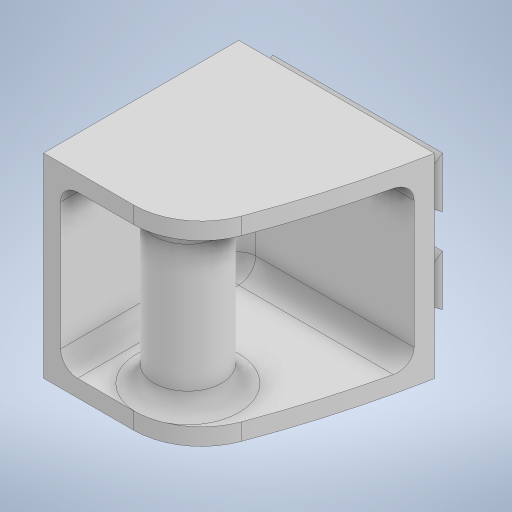
# Autodesk Inventor part: sides_fp13
Saved by Autodesk Inventor 2023 (Build 270158000, 158)
## iProperties
Created: 2023-02-13
Part Number: sides_fp13
Material: Generic
Document SubType Name: Modeling
Designer: tdal0
Density: 1 g/cm^3
Appearance: Default
Author: tdal0
Autodesk Inventor part; units mm, degrees
ref_plane "YZ Plane" through (0, 0, 0) normal (1, 0, 0) x (0, 1, 0)
ref_plane "XZ Plane" through (0, 0, 0) normal (0, 1, 0) x (-1, 0, 0)
ref_plane "XY Plane" through (0, 0, 0) normal (0, 0, 1) x (1, 0, 0)
sketch "Sketch12" plane through (0, 0, 0) normal (0, 1, 0) x (-1, 0, 0)
  line L0 (0, 0) -> (0, -102.5) construction
  line L1 (0, 0) -> (0, 102.5) construction
  line L2 (0, 102.5) -> (125, 102.5) construction
  line L3 (125, 102.5) -> (125, -102.5) construction
  line L4 (125, -102.5) -> (0, -102.5) construction
  line L5 (0, -102.5) -> (0, 102.5) construction
  line L6 (0, 102.5) -> (45, 102.5) construction
  line L7 (45, 102.5) -> (45, -102.5) construction
  line L8 (45, -102.5) -> (0, -102.5) construction
  line L9 (0, -102.5) -> (0, 102.5) construction
  line L10 (125, 0) -> (125, -217.5) construction
  line L11 (125, -217.5) -> (72.0108, -217.5) construction
  line L12 (45, -217.5) -> (45, -102.5) construction
  line L13 (125, 0) -> (125, 217.5) construction
  line L14 (125, 217.5) -> (72.0108, 217.5) construction
  line L15 (45, 217.5) -> (45, 102.5) construction
  arc A0 (34.5307, 191.4729) -> (34.5307, -191.4729) centre (548.125, 0) ccw construction
  arc A1 (34.5307, -191.4729) -> (72.0108, -217.5) centre (72.0108, -177.5) ccw construction
  arc A2 (72.0108, 217.5) -> (34.5307, 191.4729) centre (72.0108, 177.5) ccw construction
  line L16 (125, 102.5) -> (125, 107.5) construction
  line L17 (125, 217.5) -> (125, 102.5)
  line L18 (125, 102.5) -> (9.6691, 102.5)
  line L19 (125, 102.5) -> (125, 112.5) construction
  line L20 (125, 112.5) -> (11.6693, 112.5) construction
  line L21 (125, 217.5) -> (115, 217.5) construction
  line L22 (115, 217.5) -> (115, 102.5) construction
  line L23 (115, 217.5) -> (125, 217.5)
  line L24 (115, 217.5) -> (115, 112.5)
  line L25 (115, 112.5) -> (11.6693, 112.5)
  arc A3 (11.6693, 112.5) -> (9.6691, 102.5) centre (548.125, 0) ccw
  dimension "d616" = 102.5
  dimension "d617" = 102.5
  dimension "d618" = 125
  dimension "d619" = 45
  dimension "d620" = 217.5
  dimension "d621" = 217.5
  dimension "d622" = 40
  dimension "d650" = 10
  dimension "d651" = 10
  constraints: 52 end point, 13 point on circle, 12 point on line, 7 perpendicular, 4 centre point, 4 collinear, 4 parallel, 4 tangent, 3 vertical, 2 horizontal, 1 equal radius, 1 midpoint
  measures "d616" distance of L0.start L0.end
  measures "d617" distance of L0.start L1.end
  measures "d618" distance of L3.end L4.end
  measures "d619" distance of L7.end L8.end
  measures "d620" distance of L10.start L10.end
  measures "d621" distance of L10.start L13.end
  measures "d622" radius of A1
  measures "d650" distance of L2.end L19.end
  measures "d651" distance of L13.end L21.end
extrude "Extrusion12" add sketch "Sketch12" along normal blind 115
sketch "Sketch66" plane through (0, 115, 0) normal (0, 1, 0) x (1, 0, 0)
  line L0 (0, 0) -> (0, 102.5) construction
  line L1 (0, 0) -> (0, -102.5) construction
  line L2 (0, -102.5) -> (-125, -102.5) construction
  line L3 (-125, -102.5) -> (-125, 102.5) construction
  line L4 (-125, 102.5) -> (0, 102.5) construction
  line L5 (0, 102.5) -> (0, -102.5) construction
  line L6 (0, -102.5) -> (-45, -102.5) construction
  line L7 (-45, -102.5) -> (-45, 102.5) construction
  line L8 (-45, 102.5) -> (0, 102.5) construction
  line L9 (0, 102.5) -> (0, -102.5) construction
  line L10 (-125, 0) -> (-125, 217.5) construction
  line L11 (-125, 217.5) -> (-72.0108, 217.5) construction
  line L12 (-45, 217.5) -> (-45, 102.5) construction
  line L13 (-125, 0) -> (-125, -217.5) construction
  line L14 (-125, -217.5) -> (-72.0108, -217.5)
  line L15 (-45, -217.5) -> (-45, -102.5) construction
  line L16 (-120, -107.5) -> (-10.645, -107.5) construction
  arc A0 (-34.5307, -191.4729) -> (-34.5307, 191.4729) centre (-548.125, 0) ccw
  arc A1 (-72.0108, -217.5) -> (-34.5307, -191.4729) centre (-72.0108, -177.5) ccw
  arc A2 (-34.5307, 191.4729) -> (-72.0108, 217.5) centre (-72.0108, 177.5) ccw construction
  line L17 (-125, -217.5) -> (-120, -217.5) projected
  line L18 (-120, -217.5) -> (-120, -107.5)
  line L19 (-120, -217.5) -> (-120, -107.5) projected
  line L20 (-120, -107.5) -> (-10.645, -107.5)
  dimension "d643" = 102.5
  dimension "d644" = 102.5
  dimension "d645" = 125
  dimension "d646" = 45
  dimension "d647" = 217.5
  dimension "d648" = 217.5
  dimension "d649" = 40
  constraints: 36 end point, 9 point on circle, 7 perpendicular, 5 equal length, 4 point on line, 4 tangent, 3 centre point, 3 vertical, 2 horizontal, 1 equal radius, 1 midpoint
  measures "d643" distance of L0.start L0.end
  measures "d644" distance of L0.start L1.end
  measures "d645" distance of L3.end L4.end
  measures "d646" distance of L7.end L8.end
  measures "d647" distance of L10.start L10.end
  measures "d648" distance of L10.start L13.end
  measures "d649" radius of A1
extrude "Extrusion51" add sketch "Sketch66" against normal blind 10
sketch "Sketch67" plane through (0, 0, 0) normal (0, -1, 0) x (1, 0, 0)
  line L0 (-125, 217.5) -> (-72.0108, 217.5) projected
  line L1 (-120, 217.5) -> (-120, 107.5)
  arc A0 (-11.6693, 112.5) -> (-34.5307, 191.4729) centre (-548.125, 0) ccw projected
  line L2 (-120, 107.5) -> (-10.645, 107.5)
  line L3 (-120, 217.5) -> (-72.0108, 217.5)
  arc A1 (-34.5307, 191.4729) -> (-72.0108, 217.5) centre (-72.0108, 177.5) ccw projected
  arc A2 (-34.5307, 191.4729) -> (-72.0108, 217.5) centre (-72.0108, 177.5) ccw
  arc A3 (-9.6691, 102.5) -> (-10.645, 107.5) centre (-548.125, 0) ccw construction
  arc A4 (-10.645, 107.5) -> (-34.5307, 191.4729) centre (-548.125, 0) ccw
  point P0 (-105, 112.5)
  constraints: 6 end point, 4 point on circle, 2 centre point, 1 concentric, 1 perpendicular, 1 point on line, 1 vertical
extrude "Extrusion52" add sketch "Sketch67" against normal blind 10
sketch "Sketch79" plane through (0, 10, 0) normal (0, 1, 0) x (1, 0, 0)
  arc A0 (-72.0093, -220) -> (-34.5299, -193.9747) centre (-72.0093, -180) ccw construction
  circle A1 centre (-70, -187.5) radius 20
  line L0 (-120, -220) -> (-120, -107.5) projected
  line L1 (-115, -217.5) -> (-72.0108, -217.5) projected
  point P0 (0, 0)
  point P1 (-72.0093, -180)
  point P2 (-49.1947, -212.8557)
  dimension "d578" = 40
  dimension "d586" = 50
  dimension "d652" = 30
  constraints: 1 centre point, 1 coincident, 1 point on circle
  measures "d578" diameter of A1
  measures "d586" distance from line of L0 A1.centre
  measures "d652" distance from line of L1 A1.centre
extrude "Extrusion61" add sketch "Sketch79" along normal blind 95
fillet "Fillet28" radius 10 7 edges at (-63.3346, 105, 112.5) (-115, 105, 165) (-115, 57.5, 112.5) (-63.3346, 10, 112.5) (-115, 10, 165) (-90, 105, 187.5) (-90, 10, 187.5)
sketch "Sketch95" plane through (-125, 0, 102.5) normal (-1, 0, 0) x (0, 0, 1)
  line L0 (0, 0) -> (0, 115) projected
  line L1 (0, 25) -> (0, 40)
  line L2 (0, 40) -> (-10, 40)
  line L3 (0, 32.5) -> (-20, 32.5) construction
  line L4 (-20, 32.5) -> (-20, 47.5)
  line L5 (-20, 47.5) -> (-10, 40)
  line L6 (-20, 32.5) -> (-20, 17.5)
  line L7 (-20, 17.5) -> (-10, 25)
  line L8 (-10, 25) -> (0, 25)
  line L9 (0, 90) -> (0, 75)
  line L10 (0, 75) -> (-10, 75)
  line L11 (0, 82.5) -> (-20, 82.5) construction
  line L12 (-20, 82.5) -> (-20, 97.5)
  line L13 (-20, 97.5) -> (-10, 90)
  line L14 (-10, 90) -> (0, 90)
  line L15 (-20, 82.5) -> (-20, 67.5)
  line L16 (-20, 67.5) -> (-10, 75)
  line L17 (0, 0) -> (115, 0) projected
  line L18 (0, 115) -> (115, 115) projected
  point P0 (-102.5, 0)
  dimension "d631" = 15
  dimension "d632" = 10
  dimension "d633" = 20
  dimension "d634" = 15
  dimension "d635" = 15
  dimension "d636" = 15
  dimension "d637" = 20
  dimension "d638" = 15
  dimension "d639" = 15
  dimension "d653" = 25
  dimension "d654" = 25
  constraints: 32 end point, 6 point on line, 5 perpendicular, 2 horizontal, 2 midpoint, 1 parallel
  measures "d631" distance of L1.start L1.end
  measures "d632" distance of L1.end L2.end
  measures "d633" distance of L3.start L3.end
  measures "d634" distance of L3.end L4.end
  measures "d635" distance of L3.end L6.end
  measures "d636" distance of L9.start L9.end
  measures "d637" distance of L11.start L11.end
  measures "d638" distance of L11.end L12.end
  measures "d639" distance of L11.end L15.end
  measures "d653" distance between parallel lines of L17 L8
  measures "d654" distance between parallel lines of L18 L14
extrude "Extrusion64" add sketch "Sketch95" against normal blind 100
body "Solid3"
